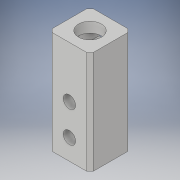
# Autodesk Inventor part: simplifiedY
Saved by Autodesk Inventor 2018 (Build 220112000, 112)
## iProperties
Created: 2020-03-14
Part Number: simplifiedY
Material: Generic
Document SubType Name: Modeling
Designer: natha
Density: 1 g/cm^3
Appearance: Default
Author: natha
Autodesk Inventor part; units mm, degrees
ref_plane "YZ Plane" through (0, 0, 0) normal (1, 0, 0) x (0, 1, 0)
ref_plane "XZ Plane" through (0, 0, 0) normal (0, 1, 0) x (-1, 0, 0)
ref_plane "XY Plane" through (0, 0, 0) normal (0, 0, 1) x (1, 0, 0)
sketch "Sketch1" plane through (0, 0, 0) normal (0, 1, 0) x (-1, 0, 0)
  line L0 (0, 0) -> (40, 0)
  line L1 (40, 0) -> (40, -40)
  line L2 (40, -40) -> (0, -40)
  line L3 (0, -40) -> (0, 0)
  dimension "d0" = 40
  dimension "d1" = 40
  constraints: 8 end point, 2 parallel, 1 horizontal, 1 perpendicular
  measures "d0" distance of L1.end L2.end
  measures "d1" distance of L0.end L1.end
extrude "Extrusion1" add sketch "Sketch1" along normal blind 100
sketch "Sketch2" plane through (-40, 0, 0) normal (0, 0, 1) x (1, 0, 0)
  circle A0 centre (20, 20) radius 6
  circle A1 centre (20, 50) radius 6
  line L0 (40, 0) -> (0, 0) projected
  line L1 (0, 0) -> (0, 100) projected
  dimension "d4" = 12
  dimension "d5" = 12
  dimension "d6" = 20
  dimension "d7" = 30
  dimension "d8" = 20
  dimension "d9" = 20
  constraints: 2 centre point
  measures "d4" diameter of A0
  measures "d5" diameter of A1
  measures "d6" distance from line of L0 A0.centre
  measures "d7" distance of A1.centre A0.centre
  measures "d8" distance from line of L1 A0.centre
  measures "d9" distance from line of L1 A1.centre
extrude "Extrusion2" cut sketch "Sketch2" against normal blind 40
sketch "Sketch3" plane through (0, 100, 0) normal (0, 1, 0) x (1, 0, 0)
  circle A0 centre (-20, 20) radius 11.15
  line L0 (-40, 40) -> (-40, 0) projected
  line L1 (-40, 0) -> (0, 0) projected
  dimension "d12" = 22.3
  dimension "d13" = 20
  dimension "d14" = 20
  constraints: 1 centre point
  measures "d12" diameter of A0
  measures "d13" distance from line of L0 A0.centre
  measures "d14" distance from line of L1 A0.centre
extrude "Extrusion3" cut sketch "Sketch3" against normal blind 30
sketch "Sketch4" plane through (0, 0, -40) normal (0, 0, -1) x (-1, 0, 0)
  line L0 (8.85, 90) -> (31.15, 90)
  line L1 (31.15, 90) -> (31.15, 80)
  line L2 (31.15, 80) -> (8.85, 80)
  line L3 (8.85, 80) -> (8.85, 90)
  line L4 (8.85, 90) -> (31.15, 80) construction
  line L5 (31.15, 90) -> (8.85, 80) construction
  line L6 (0, 0) -> (0, 100) projected
  line L7 (0, 100) -> (40, 100) projected
  point P0 (20, 85)
  dimension "d17" = 22.3
  dimension "d18" = 10
  dimension "d19" = 20
  dimension "d20" = 15
  constraints: 12 end point, 2 midpoint, 2 parallel, 1 horizontal, 1 perpendicular
  measures "d17" distance of L1.end L2.end
  measures "d18" distance of L0.end L1.end
  measures "d19" distance from line of L6 point (20, 85)
  measures "d20" distance from line of L7 point (20, 85)
extrude "Extrusion4" cut sketch "Sketch4" against normal blind 20
chamfer "Chamfer1" distance 3.175 angle 45 4 edges at (-40, 50, 0) (-40, 50, -40) (0, 50, -40) (0, 50, 0)
body "Solid1"
